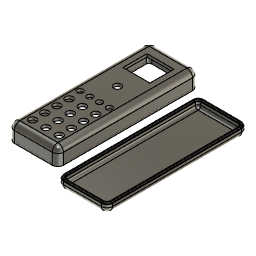
DIY Throttle Housing (Autodesk Fusion 360 design; units mm, degrees)
Autodesk Fusion 360 part; units mm, degrees
note: some values were not read from the file. Set by a fixed rule: which sketch regions a step uses.
sketch "Sketch1" plane through (0, 0, 0) normal (0, 0, 1) x (1, 0, 0)
  line L0 (0, 0) -> (127, 0)
  line L1 (127, 0) -> (127, 44.45)
  line L2 (127, 44.45) -> (0, 44.45)
  line L3 (0, 44.45) -> (0, 0)
  dimension "d1" = 127
  dimension "d18" = 44.45
  constraint horizontal L0
  constraint vertical L1
  constraint horizontal L2
  constraint vertical L3
  constraint coincident L0.start L3.end
  measures "d1" distance of L0.start L0.end
  measures "d18" distance of L0.start L2.end
extrude "Extrude1" add sketch "Sketch1" along normal blind 15.24 makes body 1
fillet "Fillet1" radius 5.08 8 edges at (63.5, 0, 0) (0, 0, 7.62) (127, 0, 7.62) (127, 22.225, 0) (127, 44.45, 7.62) (63.5, 44.45, 0) (0, 44.45, 7.62) (0, 22.225, 0) on bodies 1
shell "Shell1" thickness 2.54 removed faces 1 at (82.9733, 14.8167, 15.24) on bodies 1
sketch "Sketch2" plane through (0, 0, 15.24) normal (0, 0, 1) x (-1, 0, 0)
  arc A0 (-124.46, -39.37) -> (-121.92, -41.91) centre (-121.92, -39.37) ccw
  line L0 (-124.46, -39.37) -> (-124.46, -5.08)
  arc A1 (-121.92, -2.54) -> (-124.46, -5.08) centre (-121.92, -5.08) ccw
  line L1 (-121.92, -2.54) -> (-5.08, -2.54)
  arc A2 (-2.54, -5.08) -> (-5.08, -2.54) centre (-5.08, -5.08) ccw
  line L2 (-2.54, -5.08) -> (-2.54, -39.37)
  arc A3 (-5.08, -41.91) -> (-2.54, -39.37) centre (-5.08, -39.37) ccw
  line L3 (-5.08, -41.91) -> (-121.92, -41.91)
  arc A4 (-121.92, 0) -> (-127, -5.08) centre (-121.92, -5.08) ccw
  line L4 (-127, -5.08) -> (-127, -39.37)
  arc A5 (-127, -39.37) -> (-121.92, -44.45) centre (-121.92, -39.37) ccw
  line L5 (-121.92, -44.45) -> (-5.08, -44.45)
  arc A6 (-5.08, -44.45) -> (0, -39.37) centre (-5.08, -39.37) ccw
  line L6 (0, -39.37) -> (0, -5.08)
  arc A7 (0, -5.08) -> (-5.08, 0) centre (-5.08, -5.08) ccw
  line L7 (-5.08, 0) -> (-121.92, 0)
  line L8 (-5.08, -0.6267) -> (-121.92, -0.6267)
  arc A8 (-121.92, -0.6267) -> (-126.3733, -5.08) centre (-121.92, -5.08) ccw
  line L9 (-126.3733, -5.08) -> (-126.3733, -39.37)
  arc A9 (-126.3733, -39.37) -> (-121.92, -43.8233) centre (-121.92, -39.37) ccw
  line L10 (-121.92, -43.8233) -> (-5.08, -43.8233)
  arc A10 (-5.08, -43.8233) -> (-0.6267, -39.37) centre (-5.08, -39.37) ccw
  line L11 (-0.6267, -39.37) -> (-0.6267, -5.08)
  arc A11 (-0.6267, -5.08) -> (-5.08, -0.6267) centre (-5.08, -5.08) ccw
  arc A12 (-5.08, -42.5367) -> (-1.9133, -39.37) centre (-5.08, -39.37) ccw
  line L12 (-1.9133, -5.08) -> (-1.9133, -39.37)
  arc A13 (-1.9133, -5.08) -> (-5.08, -1.9133) centre (-5.08, -5.08) ccw
  line L13 (-121.92, -1.9133) -> (-5.08, -1.9133)
  arc A14 (-121.92, -1.9133) -> (-125.0867, -5.08) centre (-121.92, -5.08) ccw
  line L14 (-125.0867, -39.37) -> (-125.0867, -5.08)
  arc A15 (-125.0867, -39.37) -> (-121.92, -42.5367) centre (-121.92, -39.37) ccw
  line L15 (-5.08, -42.5367) -> (-121.92, -42.5367)
  dimension "d7" = -0.6267
  dimension "d8" = -0.6267
copy_body "CopyPasteBodies1" bodies 1 makes body 2
move_body "Move1" bodies 2 to x (1, 0, 0) y (0, -1, 0) z (0, 0, -1) at (0, 0, 30.48)
extrude "Extrude2" cut sketch "Sketch2" against normal blind 1.27 contours L8 A8 L9 A9 L10 A10 L11 A11 bodies 1
extrude "Extrude3" cut 1 faces at (82.9733, -0.8467, 15.24) along direction (0, 0, 1) blind 7.62 on bodies 2 bodies 2
sketch "Sketch3" plane through (0, 0, 22.86) normal (0, 0, -1) x (1, 0, 0)
  arc A0 (124.46, 39.37) -> (121.92, 41.91) centre (121.92, 39.37) ccw
  line L0 (124.46, 39.37) -> (124.46, 5.08)
  arc A1 (121.92, 2.54) -> (124.46, 5.08) centre (121.92, 5.08) ccw
  line L1 (121.92, 2.54) -> (5.08, 2.54)
  arc A2 (2.54, 5.08) -> (5.08, 2.54) centre (5.08, 5.08) ccw
  line L2 (2.54, 5.08) -> (2.54, 39.37)
  arc A3 (5.08, 41.91) -> (2.54, 39.37) centre (5.08, 39.37) ccw
  line L3 (5.08, 41.91) -> (121.92, 41.91)
  arc A4 (121.92, 0) -> (127, 5.08) centre (121.92, 5.08) ccw
  line L4 (127, 5.08) -> (127, 39.37)
  arc A5 (127, 39.37) -> (121.92, 44.45) centre (121.92, 39.37) ccw
  line L5 (121.92, 44.45) -> (5.08, 44.45)
  arc A6 (5.08, 44.45) -> (0, 39.37) centre (5.08, 39.37) ccw
  line L6 (0, 39.37) -> (0, 5.08)
  arc A7 (0, 5.08) -> (5.08, 0) centre (5.08, 5.08) ccw
  line L7 (5.08, 0) -> (121.92, 0)
  line L8 (0.762, 39.37) -> (0.762, 5.08)
  arc A8 (0.762, 5.08) -> (5.08, 0.762) centre (5.08, 5.08) ccw
  line L9 (5.08, 0.762) -> (121.92, 0.762)
  arc A9 (121.92, 0.762) -> (126.238, 5.08) centre (121.92, 5.08) ccw
  line L10 (126.238, 5.08) -> (126.238, 39.37)
  arc A10 (126.238, 39.37) -> (121.92, 43.688) centre (121.92, 39.37) ccw
  line L11 (121.92, 43.688) -> (5.08, 43.688)
  arc A11 (5.08, 43.688) -> (0.762, 39.37) centre (5.08, 39.37) ccw
  arc A12 (125.222, 39.37) -> (121.92, 42.672) centre (121.92, 39.37) ccw
  line L12 (5.08, 42.672) -> (121.92, 42.672)
  arc A13 (5.08, 42.672) -> (1.778, 39.37) centre (5.08, 39.37) ccw
  line L13 (1.778, 5.08) -> (1.778, 39.37)
  arc A14 (1.778, 5.08) -> (5.08, 1.778) centre (5.08, 5.08) ccw
  line L14 (121.92, 1.778) -> (5.08, 1.778)
  arc A15 (121.92, 1.778) -> (125.222, 5.08) centre (121.92, 5.08) ccw
  line L15 (125.222, 39.37) -> (125.222, 5.08)
  dimension "d14" = -0.762
  dimension "d15" = -0.762
extrude "Extrude4" add sketch "Sketch3" along normal blind 1.27 contours L8 A8 L9 A9 L10 A10 L11 A11 bodies 2
sketch "Sketch5" plane through (0, 0, 0) normal (0, 0, -1) x (1, 0, 0)
  line L0 (5.08, -5.08) -> (5.08, -39.37)
  line L1 (5.08, -39.37) -> (121.92, -39.37)
  line L2 (121.92, -39.37) -> (121.92, -5.08)
  line L3 (121.92, -5.08) -> (5.08, -5.08)
  line L4 (33.6067, -10.033) -> (11.9151, -10.033)
  line L5 (11.9151, -10.033) -> (11.9151, -34.417)
  line L6 (11.9151, -34.417) -> (33.6067, -34.417)
  line L7 (33.6067, -34.417) -> (33.6067, -10.033)
  line L8 (33.6067, -10.033) -> (11.9151, -34.417) construction
  line L9 (11.9151, -10.033) -> (33.6067, -34.417) construction
  line L10 (5.08, -22.225) -> (121.92, -22.225)
  circle A0 centre (49.951, -22.225) radius 3.302
  line L11 (121.92, -22.225) -> (115.57, -22.225)
  line L12 (115.57, -22.225) -> (115.57, -10.16)
  circle A1 centre (115.57, -10.16) radius 3.3655
  line L13 (49.951, -22.225) -> (66.461, -22.225)
  line L14 (66.461, -22.225) -> (66.461, -8.89)
  circle A2 centre (66.461, -8.89) radius 2.54
  point P0 (22.7609, -22.225)
  dimension "d24" = 21.6916
  dimension "d25" = 24.384
  dimension "d35" = 6.604
  dimension "d36" = 6.35
  dimension "d37" = 6.731
  dimension "d38" = 16.51
  dimension "d39" = 13.335
  dimension "d40" = 5.08
  constraint horizontal L4
  constraint perpendicular L4 L5
  constraint parallel L4 L6
  constraint parallel L5 L7
  constraint coincident L8 P0
  constraint coincident L9 P0
  constraint midpoint L0 L10.start
  constraint midpoint L2 L10.end
  constraint coincident L10 A0.centre
  constraint perpendicular L2 L11
  constraint perpendicular L11 L12
  constraint coincident L12.end A1.centre
  constraint coincident A0.centre L13.start
  constraint parallel L10 L13
  constraint perpendicular L13 L14
  constraint coincident L14.end A2.centre
  measures "d24" distance of L5.end L6.end
  measures "d25" distance of L4.end L5.end
  measures "d35" diameter of A0
  measures "d36" distance of L10.end L11.end
  measures "d37" diameter of A1
  measures "d38" distance of A0.centre L13.end
  measures "d39" distance of L13.end L14.end
  measures "d40" diameter of A2
extrude "Extrude5" cut sketch "Sketch5" against normal blind 7.62 contours L5 L6 L7 L10 | L4 L5 L7 L10 bodies 1
sketch "Sketch6" plane through (0, 0, 0) normal (0, 0, -1) x (1, 0, 0)
  line L0 (11.9151, -10.033) -> (33.6067, -10.033)
  line L1 (33.6067, -10.033) -> (33.6067, -34.417)
  line L2 (33.6067, -34.417) -> (11.9151, -34.417)
  line L3 (11.9151, -34.417) -> (11.9151, -10.033)
  line L4 (5.08, -5.08) -> (5.08, -39.37)
  line L5 (5.08, -39.37) -> (121.92, -39.37)
  line L6 (121.92, -39.37) -> (121.92, -5.08)
  line L7 (121.92, -5.08) -> (5.08, -5.08)
move_body "Move2" bodies 1 2 to x (1, 0, 0) y (0, -1, 0) z (0, 0, -1) at (0, 0, 30.48)
sketch "Sketch7" plane through (0, 0, 30.48) normal (0, 0, 1) x (-1, 0, 0)
  line L0 (-11.9151, 10.033) -> (-33.6067, 10.033)
  line L1 (-33.6067, 10.033) -> (-33.6067, 34.417)
  line L2 (-33.6067, 34.417) -> (-11.9151, 34.417)
  line L3 (-11.9151, 34.417) -> (-11.9151, 10.033)
  line L4 (-5.08, 5.08) -> (-5.08, 39.37)
  line L5 (-5.08, 39.37) -> (-121.92, 39.37)
  line L6 (-121.92, 39.37) -> (-121.92, 5.08)
  line L7 (-121.92, 5.08) -> (-5.08, 5.08)
  line L8 (-121.92, 22.225) -> (-5.08, 22.225)
  line L9 (-121.92, 22.225) -> (-115.57, 22.225)
  line L10 (-115.57, 22.225) -> (-115.57, 10.16)
  circle A0 centre (-115.57, 10.16) radius 3.3655
  dimension "d43" = 6.731
  constraint midpoint L6 L8.start
  constraint midpoint L4 L8.end
  constraint coincident L8 L9.end
  constraint perpendicular L6 L9
  constraint perpendicular L7 L10
  constraint coincident L10.end A0.centre
  measures "d43" diameter of A0
extrude "Extrude7" cut sketch "Sketch7" against normal through all contours A0 bodies 1
pattern_linear "R-Pattern1" count 3 spacing 12.065 along (0, -1, 0) count 4 spacing 11.0067 along (-1, 0, 0) of "Extrude7"
sketch "Sketch8" plane through (0, 0, 30.48) normal (0, 0, 1) x (-1, 0, 0)
  circle A0 centre (-50.8, 22.225) radius 12.7
  circle A1 centre (-50.8, 22.225) radius 3.3655
  line L0 (-79.1849, 22.225) -> (-63.5, 22.225)
  line L1 (-71.3425, 22.225) -> (-71.3425, 9.015)
  circle A2 centre (-71.3425, 9.015) radius 2.667
  dimension "d49" = 25.4
  dimension "d50" = 6.731
  dimension "d51" = 5.334
  constraint concentric A0 A1
  constraint coincident A0 L0.end
  constraint horizontal L0
  constraint midpoint L0 L1.start
  constraint coincident L1.end A2.centre
  measures "d49" diameter of A0
  measures "d50" diameter of A1
  measures "d51" diameter of A2
extrude "Extrude8" cut sketch "Sketch8" against normal blind 5.08 contours A1 bodies 1
extrude "Extrude9" cut sketch "Sketch8" against normal blind 2.54 contours A2 bodies 1
pattern_linear "R-Pattern2" count 4 spacing 8.8053 along (0, -1, 0) of "Extrude9"
move_body "Move3" bodies 2 1 to x (0, -1, 0) y (1, 0, 0) z (0, 0, 1) at (0, 0, 0)
equation "d48 = 0.975 * 1.33333333 in"
named bodies: "Top", "Bottom"
